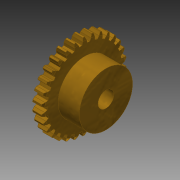
# Autodesk Inventor part: Zahnrad Messing z30
Saved by Autodesk Inventor 2017.3 (Build 213256000, 256)
## iProperties
Category: PARTsolutions
Company: MAEDLER
Created: 2018-08-20
Part Number: Zahnrad Messing z30
Material: Messing, weicher Gelbton, geschweißt
Catalog Web Link: www.cadenas.de
Description: Stzr Messing Ms58-Spur Gears, Brass, Helical Tooth Right Hand, with one-sided hub
Vendor: MAEDLER
Document SubType Name: Modeling
Designer: psadmin
Manufacturer: MAEDLER
Mass: 5.2 g
Surface Area: 6.86122 cm^2
Volume: 0.619705 cm^3
Density: 8.39109 g/cm^3
Appearance: Schweißnaht - Messing
PSOL_IDENT_0: {$CADENAS_DATA\23d-libs\maedler\antriebselemente\stirnzahnraeder\stirnzahnraeder_messing\stzr_messin
PSOL_IDENT_1: g_ms58.prj},204 {VTYP=3D},{NB=Stzr Messing Ms58 26103000},{LINA=Stzr Messing Ms58 26103000},{NN=Stzr
PSOL_IDENT_2: Messing Ms58},{DATE=03.08.2018 09:08:56},{GEOMDATE=26.07.2018 09:15:44},{VERSION=},{LINEID=360},{WB
PSOL_IDENT_3: VAR=},{WBNUMERIC=}  {NB=Stzr Messing Ms58 26103000},{LINA=Stzr Messing Ms58 26103000},{KT=DUMMY},{AR
PSOL_IDENT_4: TNR=26103000},{WST=Messing (Ms58)},{M=0.5},{Z=30},{PDF=PDF Katalogseite},{B1=2.0},{DA=16.00},{D=15.0
PSOL_IDENT_5: 0},{NL=4},{ND=10},{B=3.00},{MD=3.0},{GEW=5.200}
NN: Stzr Messing Ms58
NT: Spur Gears, Brass, Helical Tooth Right Hand, with one-sided hub
NB: Stzr Messing Ms58 26103000
NBSYN: Stzr Messing Ms58 $ARTNR.
LINA: Stzr Messing Ms58 26103000
ARTNR: 26103000
WST: Messing (Ms58)
M: 0.5
Z: 30
PDF: PDF Katalogseite
B1: 2
DA: 16
D: 15
NL: 4
ND: 10
B: 3
MD: 3
GEW: 5.2
SUPPLIER: MAEDLER
ARTICLENO: Stzr Messing Ms58 26103000
BOMINFO: Stzr Messing Ms58 26103000
CREATOR: CADENAS GmbH
Title: Stzr Messing Ms58 26103000
Author: Cadenas PARTsolutions
Comments: Spur Gears, Brass, Helical Tooth Right Hand, with one-sided hub
Autodesk Inventor part; units mm, degrees
ref_plane "YZ Plane" through (0, 0, 0) normal (1, 0, 0) x (0, 1, 0)
ref_plane "XZ Plane" through (0, 0, 0) normal (0, 1, 0) x (-1, 0, 0)
ref_plane "XY Plane" through (0, 0, 0) normal (0, 0, 1) x (1, 0, 0)
sketch "Skizze_1" plane through (0, 0, 0) normal (0, 0, 1) x (1, 0, 0)
  line L0 (6, 0) -> (0, 0)
  line L1 (0, 1.5) -> (6, 1.5)
  line L2 (6, 1.5) -> (6, 5)
  line L3 (6, 5) -> (2, 5)
  line L4 (2, 5) -> (2, 7.5)
  line L5 (2, 7.5) -> (1, 10.2475)
  line L6 (1, 10.2475) -> (0, 7.5)
  line L7 (0, 7.5) -> (0, 1.5)
  constraints: 16 end point
revolve "Revolution1" add sketch "Skizze_1" angle 360 about axis through (6, 0, 0) along (1, 0, 0)
sketch "Skizze_2" plane through (2, 0, 0) normal (1, 0, 0) x (0, 0, -1)
  circle A0 centre (0, 0) radius 24
  arc A1 (-7.9983, 0.1667) -> (-7.9983, -0.1667) centre (0, 0) ccw
  line L0 (-7.9983, -0.1667) -> (-7.4913, -0.3616)
  line L1 (-7.4913, -0.3616) -> (-6.9829, -0.4883)
  arc A2 (-6.9829, -0.4883) -> (-6.9319, -0.9742) centre (0, 0) ccw
  line L2 (-6.9319, -0.9742) -> (-7.4027, -1.2039)
  line L3 (-7.4027, -1.2039) -> (-7.8581, -1.4999)
  arc A3 (-7.8581, -1.4999) -> (-7.7888, -1.826) centre (0, 0) ccw
  line L4 (-7.7888, -1.826) -> (-7.2524, -1.9112)
  line L5 (-7.2524, -1.9112) -> (-6.7288, -1.9295)
  arc A4 (-6.7288, -1.9295) -> (-6.5778, -2.3941) centre (0, 0) ccw
  line L6 (-6.5778, -2.3941) -> (-6.9907, -2.7167)
  line L7 (-6.9907, -2.7167) -> (-7.3746, -3.1009)
  arc A5 (-7.3746, -3.1009) -> (-7.239, -3.4054) centre (0, 0) ccw
  line L8 (-7.239, -3.4054) -> (-6.6966, -3.3773)
  line L9 (-6.6966, -3.3773) -> (-6.1806, -3.2863)
  arc A6 (-6.1806, -3.2863) -> (-5.9363, -3.7094) centre (0, 0) ccw
  line L10 (-5.9363, -3.7094) -> (-6.2731, -4.1108)
  line L11 (-6.2731, -4.1108) -> (-6.5687, -4.5664)
  arc A7 (-6.5687, -4.5664) -> (-6.3728, -4.8361) centre (0, 0) ccw
  line L12 (-6.3728, -4.8361) -> (-5.8481, -4.6958)
  line L13 (-5.8481, -4.6958) -> (-5.3623, -4.4995)
  arc A8 (-5.3623, -4.4995) -> (-5.0354, -4.8626) centre (0, 0) ccw
  line L14 (-5.0354, -4.8626) -> (-5.2813, -5.3252)
  line L15 (-5.2813, -5.3252) -> (-5.4757, -5.8323)
  arc A9 (-5.4757, -5.8323) -> (-5.228, -6.0554) centre (0, 0) ccw
  line L16 (-5.228, -6.0554) -> (-4.744, -5.809)
  line L17 (-4.744, -5.809) -> (-4.3096, -5.5161)
  arc A10 (-4.3096, -5.5161) -> (-3.9144, -5.8033) centre (0, 0) ccw
  line L18 (-3.9144, -5.8033) -> (-4.0588, -6.3069)
  line L19 (-4.0588, -6.3069) -> (-4.1435, -6.8434)
  arc A11 (-4.1435, -6.8434) -> (-3.8548, -7.01) centre (0, 0) ccw
  line L20 (-3.8548, -7.01) -> (-3.4325, -6.6684)
  line L21 (-3.4325, -6.6684) -> (-3.0686, -6.2916)
  arc A12 (-3.0686, -6.2916) -> (-2.6222, -6.4903) centre (0, 0) ccw
  line L22 (-2.6222, -6.4903) -> (-2.6588, -7.0129)
  line L23 (-2.6588, -7.0129) -> (-2.6301, -7.5553)
  arc A13 (-2.6301, -7.5553) -> (-2.3131, -7.6583) centre (0, 0) ccw
  line L24 (-2.3131, -7.6583) -> (-1.9711, -7.2364)
  line L25 (-1.9711, -7.2364) -> (-1.6935, -6.7921)
  arc A14 (-1.6935, -6.7921) -> (-1.2155, -6.8937) centre (0, 0) ccw
  line L26 (-1.2155, -6.8937) -> (-1.1426, -7.4124)
  line L27 (-1.1426, -7.4124) -> (-1.0018, -7.937)
  arc A15 (-1.0018, -7.937) -> (-0.6703, -7.9719) centre (0, 0) ccw
  line L28 (-0.6703, -7.9719) -> (-0.4235, -7.488)
  line L29 (-0.4235, -7.488) -> (-0.2443, -6.9957)
  arc A16 (-0.2443, -6.9957) -> (0.2443, -6.9957) centre (0, 0) ccw
  line L30 (0.2443, -6.9957) -> (0.4235, -7.488)
  line L31 (0.4235, -7.488) -> (0.6703, -7.9719)
  arc A17 (0.6703, -7.9719) -> (1.0018, -7.937) centre (0, 0) ccw
  line L32 (1.0018, -7.937) -> (1.1426, -7.4124)
  line L33 (1.1426, -7.4124) -> (1.2155, -6.8937)
  arc A18 (1.2155, -6.8937) -> (1.6935, -6.7921) centre (0, 0) ccw
  line L34 (1.6935, -6.7921) -> (1.9711, -7.2364)
  line L35 (1.9711, -7.2364) -> (2.3131, -7.6583)
  arc A19 (2.3131, -7.6583) -> (2.6301, -7.5553) centre (0, 0) ccw
  line L36 (2.6301, -7.5553) -> (2.6588, -7.0129)
  line L37 (2.6588, -7.0129) -> (2.6222, -6.4903)
  arc A20 (2.6222, -6.4903) -> (3.0686, -6.2916) centre (0, 0) ccw
  line L38 (3.0686, -6.2916) -> (3.4325, -6.6684)
  line L39 (3.4325, -6.6684) -> (3.8548, -7.01)
  arc A21 (3.8548, -7.01) -> (4.1435, -6.8434) centre (0, 0) ccw
  line L40 (4.1435, -6.8434) -> (4.0588, -6.3069)
  line L41 (4.0588, -6.3069) -> (3.9144, -5.8033)
  arc A22 (3.9144, -5.8033) -> (4.3096, -5.5161) centre (0, 0) ccw
  line L42 (4.3096, -5.5161) -> (4.744, -5.809)
  line L43 (4.744, -5.809) -> (5.228, -6.0554)
  arc A23 (5.228, -6.0554) -> (5.4757, -5.8323) centre (0, 0) ccw
  line L44 (5.4757, -5.8323) -> (5.2813, -5.3252)
  line L45 (5.2813, -5.3252) -> (5.0354, -4.8626)
  arc A24 (5.0354, -4.8626) -> (5.3623, -4.4995) centre (0, 0) ccw
  line L46 (5.3623, -4.4995) -> (5.8481, -4.6958)
  line L47 (5.8481, -4.6958) -> (6.3728, -4.8361)
  arc A25 (6.3728, -4.8361) -> (6.5687, -4.5664) centre (0, 0) ccw
  line L48 (6.5687, -4.5664) -> (6.2731, -4.1108)
  line L49 (6.2731, -4.1108) -> (5.9363, -3.7094)
  arc A26 (5.9363, -3.7094) -> (6.1806, -3.2863) centre (0, 0) ccw
  line L50 (6.1806, -3.2863) -> (6.6966, -3.3773)
  line L51 (6.6966, -3.3773) -> (7.239, -3.4054)
  arc A27 (7.239, -3.4054) -> (7.3746, -3.1009) centre (0, 0) ccw
  line L52 (7.3746, -3.1009) -> (6.9907, -2.7167)
  line L53 (6.9907, -2.7167) -> (6.5778, -2.3941)
  arc A28 (6.5778, -2.3941) -> (6.7288, -1.9295) centre (0, 0) ccw
  line L54 (6.7288, -1.9295) -> (7.2524, -1.9112)
  line L55 (7.2524, -1.9112) -> (7.7888, -1.826)
  arc A29 (7.7888, -1.826) -> (7.8581, -1.4999) centre (0, 0) ccw
  line L56 (7.8581, -1.4999) -> (7.4027, -1.2039)
  line L57 (7.4027, -1.2039) -> (6.9319, -0.9742)
  arc A30 (6.9319, -0.9742) -> (6.9829, -0.4883) centre (0, 0) ccw
  line L58 (6.9829, -0.4883) -> (7.4913, -0.3616)
  line L59 (7.4913, -0.3616) -> (7.9983, -0.1667)
  arc A31 (7.9983, -0.1667) -> (7.9983, 0.1667) centre (0, 0) ccw
  line L60 (7.9983, 0.1667) -> (7.4913, 0.3616)
  line L61 (7.4913, 0.3616) -> (6.9829, 0.4883)
  arc A32 (6.9829, 0.4883) -> (6.9319, 0.9742) centre (0, 0) ccw
  line L62 (6.9319, 0.9742) -> (7.4027, 1.2039)
  line L63 (7.4027, 1.2039) -> (7.8581, 1.4999)
  arc A33 (7.8581, 1.4999) -> (7.7888, 1.826) centre (0, 0) ccw
  line L64 (7.7888, 1.826) -> (7.2524, 1.9112)
  line L65 (7.2524, 1.9112) -> (6.7288, 1.9295)
  arc A34 (6.7288, 1.9295) -> (6.5778, 2.3941) centre (0, 0) ccw
  line L66 (6.5778, 2.3941) -> (6.9907, 2.7167)
  line L67 (6.9907, 2.7167) -> (7.3746, 3.1009)
  arc A35 (7.3746, 3.1009) -> (7.239, 3.4054) centre (0, 0) ccw
  line L68 (7.239, 3.4054) -> (6.6966, 3.3773)
  line L69 (6.6966, 3.3773) -> (6.1806, 3.2863)
  arc A36 (6.1806, 3.2863) -> (5.9363, 3.7094) centre (0, 0) ccw
  line L70 (5.9363, 3.7094) -> (6.2731, 4.1108)
  line L71 (6.2731, 4.1108) -> (6.5687, 4.5664)
  arc A37 (6.5687, 4.5664) -> (6.3728, 4.8361) centre (0, 0) ccw
  line L72 (6.3728, 4.8361) -> (5.8481, 4.6958)
  line L73 (5.8481, 4.6958) -> (5.3623, 4.4995)
  arc A38 (5.3623, 4.4995) -> (5.0354, 4.8626) centre (0, 0) ccw
  line L74 (5.0354, 4.8626) -> (5.2813, 5.3252)
  line L75 (5.2813, 5.3252) -> (5.4757, 5.8323)
  arc A39 (5.4757, 5.8323) -> (5.228, 6.0554) centre (0, 0) ccw
  line L76 (5.228, 6.0554) -> (4.744, 5.809)
  line L77 (4.744, 5.809) -> (4.3096, 5.5161)
  arc A40 (4.3096, 5.5161) -> (3.9144, 5.8033) centre (0, 0) ccw
  line L78 (3.9144, 5.8033) -> (4.0588, 6.3069)
  line L79 (4.0588, 6.3069) -> (4.1435, 6.8434)
  arc A41 (4.1435, 6.8434) -> (3.8548, 7.01) centre (0, 0) ccw
  line L80 (3.8548, 7.01) -> (3.4325, 6.6684)
  line L81 (3.4325, 6.6684) -> (3.0686, 6.2916)
  arc A42 (3.0686, 6.2916) -> (2.6222, 6.4903) centre (0, 0) ccw
  line L82 (2.6222, 6.4903) -> (2.6588, 7.0129)
  line L83 (2.6588, 7.0129) -> (2.6301, 7.5553)
  arc A43 (2.6301, 7.5553) -> (2.3131, 7.6583) centre (0, 0) ccw
  line L84 (2.3131, 7.6583) -> (1.9711, 7.2364)
  line L85 (1.9711, 7.2364) -> (1.6935, 6.7921)
  arc A44 (1.6935, 6.7921) -> (1.2155, 6.8937) centre (0, 0) ccw
  line L86 (1.2155, 6.8937) -> (1.1426, 7.4124)
  line L87 (1.1426, 7.4124) -> (1.0018, 7.937)
  arc A45 (1.0018, 7.937) -> (0.6703, 7.9719) centre (0, 0) ccw
  line L88 (0.6703, 7.9719) -> (0.4235, 7.488)
  line L89 (0.4235, 7.488) -> (0.2443, 6.9957)
  arc A46 (0.2443, 6.9957) -> (-0.2443, 6.9957) centre (0, 0) ccw
  line L90 (-0.2443, 6.9957) -> (-0.4235, 7.488)
  line L91 (-0.4235, 7.488) -> (-0.6703, 7.9719)
  arc A47 (-0.6703, 7.9719) -> (-1.0018, 7.937) centre (0, 0) ccw
  line L92 (-1.0018, 7.937) -> (-1.1426, 7.4124)
  line L93 (-1.1426, 7.4124) -> (-1.2155, 6.8937)
  arc A48 (-1.2155, 6.8937) -> (-1.6935, 6.7921) centre (0, 0) ccw
  line L94 (-1.6935, 6.7921) -> (-1.9711, 7.2364)
  line L95 (-1.9711, 7.2364) -> (-2.3131, 7.6583)
  arc A49 (-2.3131, 7.6583) -> (-2.6301, 7.5553) centre (0, 0) ccw
  line L96 (-2.6301, 7.5553) -> (-2.6588, 7.0129)
  line L97 (-2.6588, 7.0129) -> (-2.6222, 6.4903)
  arc A50 (-2.6222, 6.4903) -> (-3.0686, 6.2916) centre (0, 0) ccw
  line L98 (-3.0686, 6.2916) -> (-3.4325, 6.6684)
  line L99 (-3.4325, 6.6684) -> (-3.8548, 7.01)
  arc A51 (-3.8548, 7.01) -> (-4.1435, 6.8434) centre (0, 0) ccw
  line L100 (-4.1435, 6.8434) -> (-4.0588, 6.3069)
  line L101 (-4.0588, 6.3069) -> (-3.9144, 5.8033)
  arc A52 (-3.9144, 5.8033) -> (-4.3096, 5.5161) centre (0, 0) ccw
  line L102 (-4.3096, 5.5161) -> (-4.744, 5.809)
  line L103 (-4.744, 5.809) -> (-5.228, 6.0554)
  arc A53 (-5.228, 6.0554) -> (-5.4757, 5.8323) centre (0, 0) ccw
  line L104 (-5.4757, 5.8323) -> (-5.2813, 5.3252)
  line L105 (-5.2813, 5.3252) -> (-5.0354, 4.8626)
  arc A54 (-5.0354, 4.8626) -> (-5.3623, 4.4995) centre (0, 0) ccw
  line L106 (-5.3623, 4.4995) -> (-5.8481, 4.6958)
  line L107 (-5.8481, 4.6958) -> (-6.3728, 4.8361)
  arc A55 (-6.3728, 4.8361) -> (-6.5687, 4.5664) centre (0, 0) ccw
  line L108 (-6.5687, 4.5664) -> (-6.2731, 4.1108)
  line L109 (-6.2731, 4.1108) -> (-5.9363, 3.7094)
  arc A56 (-5.9363, 3.7094) -> (-6.1806, 3.2863) centre (0, 0) ccw
  line L110 (-6.1806, 3.2863) -> (-6.6966, 3.3773)
  line L111 (-6.6966, 3.3773) -> (-7.239, 3.4054)
  arc A57 (-7.239, 3.4054) -> (-7.3746, 3.1009) centre (0, 0) ccw
  line L112 (-7.3746, 3.1009) -> (-6.9907, 2.7167)
  line L113 (-6.9907, 2.7167) -> (-6.5778, 2.3941)
  arc A58 (-6.5778, 2.3941) -> (-6.7288, 1.9295) centre (0, 0) ccw
  line L114 (-6.7288, 1.9295) -> (-7.2524, 1.9112)
  line L115 (-7.2524, 1.9112) -> (-7.7888, 1.826)
  arc A59 (-7.7888, 1.826) -> (-7.8581, 1.4999) centre (0, 0) ccw
  line L116 (-7.8581, 1.4999) -> (-7.4027, 1.2039)
  line L117 (-7.4027, 1.2039) -> (-6.9319, 0.9742)
  arc A60 (-6.9319, 0.9742) -> (-6.9829, 0.4883) centre (0, 0) ccw
  line L118 (-6.9829, 0.4883) -> (-7.4913, 0.3616)
  line L119 (-7.4913, 0.3616) -> (-7.9983, 0.1667)
  constraints: 240 end point, 120 point on circle, 61 centre point
extrude "Extrusion1" cut sketch "Skizze_2" along normal mid plane 12
body "Solid1"
